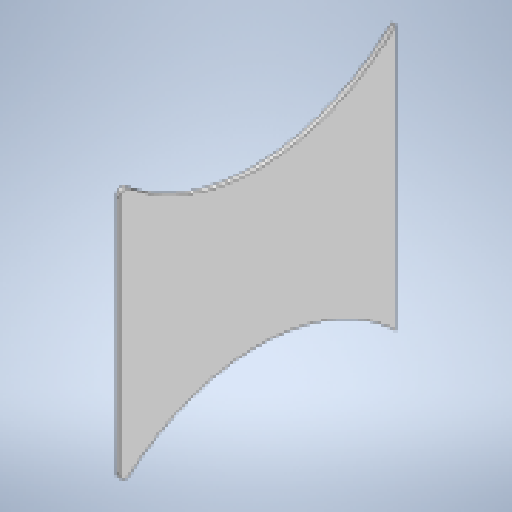
# Autodesk Inventor part: грань тела
Saved by Autodesk Inventor 2023.1 (Build 271208000, 208)
## iProperties
Created: 2024-11-21
Part Number: грань тела
Material: Типовые
Document SubType Name: Modeling
Designer: DELL
Density: 1 g/cm^3
Appearance: По умолчанию
Author: DELL
Autodesk Inventor part; units mm, degrees
ref_plane "YZ Plane" through (0, 0, 0) normal (1, 0, 0) x (0, 1, 0)
ref_plane "XZ Plane" through (0, 0, 0) normal (0, 1, 0) x (-1, 0, 0)
ref_plane "XY Plane" through (0, 0, 0) normal (0, 0, 1) x (1, 0, 0)
sketch "Эскиз1" plane through (0, 0, 0) normal (0, 0, 1) x (1, 0, 0)
  line L0 (2, -120) -> (-2, -120)
  line L1 (-2, -120) -> (-2, 120)
  line L2 (-2, 120) -> (2, 120)
  line L3 (2, 120) -> (2, -120)
  line L4 (2, -120) -> (-2, 120) construction
  line L5 (-2, -120) -> (2, 120) construction
  point P0 (0, 0)
  dimension "d0" = 4
  dimension "d1" = 240
  constraints: 12 end point, 2 midpoint, 2 parallel, 1 horizontal, 1 perpendicular
  measures "d0" distance of L1.end L2.end
  measures "d1" distance of L0.end L1.end
extrude "Выдавливание1" add sketch "Эскиз1" along normal blind 250
sketch "Эскиз3" plane through (2, -120, 0) normal (1, 0, 0) x (0, 0, -1)
  line L0 (0, 0) -> (0, 240) construction
  line L1 (0, 240) -> (-250, 240) construction
  line L2 (-250, 0) -> (-250, 240) construction
  line L3 (0, 0) -> (-250, 0) construction
  line L4 (-250, 240) -> (-250, 0) construction
  line L5 (-250, 0) -> (0, 240) construction
  line L6 (0, 120) -> (-250, 120) construction
  line L7 (0, 240) -> (-250, 240) projected
  arc A0 (-250, 240) -> (0, 240) centre (-125, 369.2971) ccw
  arc A1 (0, 0) -> (-250, 0) centre (-125, -129.2971) ccw
  line L8 (-250, 0) -> (0, 0)
  constraints: 6 end point, 4 point on circle, 2 centre point, 1 midpoint, 1 perpendicular, 1 symmetric about line, 1 other
extrude "Выдавливание2" cut sketch "Эскиз3" against normal blind 4
fillet "Сопряжение1" radius 5 1 edges at (0, 120, 250)
fillet "Сопряжение2" radius 5 1 edges at (0, -120, 250)
